Autodesk Fusion 360 part; units mm, degrees
(part 2 of 2)
fillet "Fillet2'" radius 0.5 4 edges at (74.2484, -13.991, 0.5) (60.2372, 0.0024, 0.5) (74.2484, 14.009, 0.5) (88.2372, 0.0024, 0.5) on bodies 7 in component "guards"
sketch "Sketch11" plane through (0, 0, 6) normal (0, 0, 1) x (-1, 0, 0)
  line L0 (-41.1231, -44.3731) -> (-33.1231, -44.3731)
  arc A0 (-33.1231, -45.8731) -> (-33.1231, -44.3731) centre (-33.1231, -45.1231) ccw
  line L1 (-33.1231, -45.8731) -> (-41.1231, -45.8731)
  arc A1 (-41.1231, -44.3731) -> (-41.1231, -45.8731) centre (-41.1231, -45.1231) ccw
  line L2 (-43.8731, -42.1231) -> (-43.8731, -32.1231)
  arc A2 (-42.3731, -32.1231) -> (-43.8731, -32.1231) centre (-43.1231, -32.1231) ccw
  line L3 (-42.3731, -32.1231) -> (-42.3731, -42.1231)
  arc A3 (-43.8731, -42.1231) -> (-42.3731, -42.1231) centre (-43.1231, -42.1231) ccw
  line L4 (-31.8731, -42.1231) -> (-31.8731, -32.1231)
  arc A4 (-30.3731, -32.1231) -> (-31.8731, -32.1231) centre (-31.1231, -32.1231) ccw
  line L5 (-30.3731, -32.1231) -> (-30.3731, -42.1231)
  arc A5 (-31.8731, -42.1231) -> (-30.3731, -42.1231) centre (-31.1231, -42.1231) ccw
  line L6 (-41.1231, -28.3731) -> (-33.1231, -28.3731)
  arc A6 (-33.1231, -29.8731) -> (-33.1231, -28.3731) centre (-33.1231, -29.1231) ccw
  line L7 (-33.1231, -29.8731) -> (-41.1231, -29.8731)
  arc A7 (-41.1231, -28.3731) -> (-41.1231, -29.8731) centre (-41.1231, -29.1231) ccw
  circle A8 centre (-45, -29.2462) radius 0.75
  circle A9 centre (-23.2462, -30.2462) radius 0.75
  circle A10 centre (-23.2462, -51) radius 0.75
  circle A11 centre (-51, -51) radius 0.75
  circle A12 centre (-45, -45) radius 0.75
  circle A13 centre (-23.2462, -44) radius 0.75
  circle A14 centre (-23.2462, -23.2462) radius 0.75
  circle A15 centre (-51, -30.2462) radius 0.75
  circle A16 centre (-44, -23.2462) radius 0.75
  circle A17 centre (-29.2462, -29.2462) radius 0.75
  circle A18 centre (-30.2462, -51) radius 0.75
  circle A19 centre (-51, -44) radius 0.75
  circle A20 centre (-44, -51) radius 0.75
  circle A21 centre (-29.2462, -45) radius 0.75
  circle A22 centre (-30.2462, -23.2462) radius 0.75
  circle A23 centre (-51, -23.2462) radius 0.75
  line L8 (-53.3731, -53.3731) -> (-20.8731, -53.3731)
  line L9 (-20.8731, -53.3731) -> (-20.8731, -20.8731)
  line L10 (-20.8731, -20.8731) -> (-53.3731, -20.8731)
  line L11 (-53.3731, -20.8731) -> (-53.3731, -53.3731)
  circle A24 centre (-51, -23.2462) radius 0.75
  circle A25 centre (-51, -51) radius 0.75
  circle A26 centre (-23.2462, -51) radius 0.75
  circle A27 centre (-23.2462, -23.2462) radius 0.75
  circle A28 centre (-23.2462, -23.2462) radius 1.5
  circle A29 centre (-51, -23.2462) radius 1.5
  circle A30 centre (-51, -51) radius 1.5
  circle A31 centre (-23.2462, -51) radius 1.5
  dimension "d111" = 3
  dimension "d112" = 3
  dimension "d113" = 3
  dimension "d114" = 3
  constraint concentric A23 A24
  constraint concentric A11 A25
  constraint concentric A10 A26
  constraint concentric A14 A27
  constraint concentric A27 A28
  constraint concentric A24 A29
  constraint concentric A25 A30
  constraint concentric A26 A31
  measures "d111" diameter of A28
  measures "d112" diameter of A29
  measures "d113" diameter of A30
  measures "d114" diameter of A31
extrude "Extrude1'''" add sketch "Sketch11" along normal blind 2 from surface at 10 separate body contours A8 | A9 | A12 | A13 | A15 | A16 | A17 | A18 | A19 | A20 | A21 | A22 | L8 L9 L10 L11 makes body 8 in component "platform2"
extrude "Extrude2'''" add sketch "Sketch11" along normal blind 1 from surface at 10 contours A28 | A29 | A30 | A31 bodies 8 in component "platform2"
extrude "Extrude1''''" add sketch "Sketch11" along normal blind 10 separate body contours A28 | A29 | A30 | A31 makes body 9 at (51.6843, 24.581, 9.3333) makes body 10 at (49.6827, 50.2826, 9.3333) makes body 11 at (21.7481, 23.321, 12.6667) makes body 12 at (21.9289, 50.2826, 9.3333) in component "posts"
sketch "Sketch12" plane through (0, 0, 18) normal (0, 0, 1) x (-1, 0, 0)
  arc A0 (-33.1231, -29.8731) -> (-33.1231, -28.3731) centre (-33.1231, -29.1231) ccw
  line L0 (-33.1231, -29.8731) -> (-41.1231, -29.8731)
  arc A1 (-41.1231, -28.3731) -> (-41.1231, -29.8731) centre (-41.1231, -29.1231) ccw
  line L1 (-41.1231, -28.3731) -> (-33.1231, -28.3731)
  arc A2 (-30.3731, -32.1231) -> (-31.8731, -32.1231) centre (-31.1231, -32.1231) ccw
  line L2 (-30.3731, -32.1231) -> (-30.3731, -42.1231)
  arc A3 (-31.8731, -42.1231) -> (-30.3731, -42.1231) centre (-31.1231, -42.1231) ccw
  line L3 (-31.8731, -42.1231) -> (-31.8731, -32.1231)
  arc A4 (-33.1231, -45.8731) -> (-33.1231, -44.3731) centre (-33.1231, -45.1231) ccw
  line L4 (-33.1231, -45.8731) -> (-41.1231, -45.8731)
  arc A5 (-41.1231, -44.3731) -> (-41.1231, -45.8731) centre (-41.1231, -45.1231) ccw
  line L5 (-41.1231, -44.3731) -> (-33.1231, -44.3731)
  arc A6 (-42.3731, -32.1231) -> (-43.8731, -32.1231) centre (-43.1231, -32.1231) ccw
  line L6 (-42.3731, -32.1231) -> (-42.3731, -42.1231)
  arc A7 (-43.8731, -42.1231) -> (-42.3731, -42.1231) centre (-43.1231, -42.1231) ccw
  line L7 (-43.8731, -42.1231) -> (-43.8731, -32.1231)
  circle A8 centre (-23.2462, -51) radius 1.5
  circle A9 centre (-23.2462, -23.2462) radius 1.5
  circle A10 centre (-51, -51) radius 1.5
  circle A11 centre (-51, -23.2462) radius 1.5
  line L8 (-53.3731, -20.8731) -> (-53.3731, -53.3731)
  line L9 (-53.3731, -53.3731) -> (-20.8731, -53.3731)
  line L10 (-20.8731, -53.3731) -> (-20.8731, -20.8731)
  line L11 (-20.8731, -20.8731) -> (-53.3731, -20.8731)
  line L12 (-41.1231, -23.9962) -> (-33.1231, -23.9962)
  arc A12 (-33.1231, -23.9962) -> (-33.1231, -22.4962) centre (-33.1231, -23.2462) ccw
  line L13 (-33.1231, -22.4962) -> (-41.1231, -22.4962)
  arc A13 (-41.1231, -22.4962) -> (-41.1231, -23.9962) centre (-41.1231, -23.2462) ccw
  line L14 (-41.1231, -23.2462) -> (-33.1231, -23.2462) construction
  line L15 (-51, -23.2462) -> (-51, -51)
  line L16 (-23.2462, -23.2462) -> (-23.2462, -51)
  line L17 (-48.5, -45.1231) -> (-48.5, -29.1231)
  arc A14 (-48.5, -29.1231) -> (-53.5, -29.1231) centre (-51, -29.1231) ccw
  line L18 (-53.5, -29.1231) -> (-53.5, -45.1231)
  arc A15 (-53.5, -45.1231) -> (-48.5, -45.1231) centre (-51, -45.1231) ccw
  line L19 (-51, -45.1231) -> (-51, -29.1231) construction
  line L20 (-20.7462, -45.1231) -> (-20.7462, -29.1231)
  arc A16 (-20.7462, -29.1231) -> (-25.7462, -29.1231) centre (-23.2462, -29.1231) ccw
  line L21 (-25.7462, -29.1231) -> (-25.7462, -45.1231)
  arc A17 (-25.7462, -45.1231) -> (-20.7462, -45.1231) centre (-23.2462, -45.1231) ccw
  line L22 (-23.2462, -45.1231) -> (-23.2462, -29.1231) construction
  line L23 (-23.2462, -47.6231) -> (-20.8731, -47.6231)
  line L24 (-23.2462, -26.6231) -> (-20.8731, -26.6231)
  line L25 (-51, -26.6231) -> (-53.3731, -26.6231)
  line L26 (-51, -47.6231) -> (-53.3731, -47.6231)
  line L27 (-37.1231, -32.5) -> (-36.5, -35)
  line L28 (-37.1231, -32.5) -> (-37.7462, -35)
  line L29 (-37.7462, -35) -> (-37.1231, -35)
  line L30 (-36.5, -35) -> (-37.1231, -35)
  point P0 (-51, -37.1231)
  point P1 (-23.2462, -37.1231)
  dimension "d125" = 1.5
  dimension "d126" = 5
  dimension "d127" = 5
  constraint tangent L12 A12
  constraint tangent A12 L13
  constraint parallel L12 L13
  constraint tangent L13 A13
  constraint tangent L12 A13
  constraint coincident A11.centre L15.start
  constraint coincident A10.centre L15.end
  constraint coincident A9.centre L16.start
  constraint coincident A8.centre L16.end
  constraint tangent L17 A14
  constraint tangent A14 L18
  constraint parallel L17 L18
  constraint tangent L18 A15
  constraint tangent L17 A15
  constraint parallel L15 L19
  constraint midpoint L15 P0
  constraint midpoint L19 P0
  constraint tangent L20 A16
  constraint tangent A16 L21
  constraint parallel L20 L21
  constraint tangent L21 A17
  constraint tangent L20 A17
  constraint parallel L16 L22
  constraint midpoint L16 P1
  constraint midpoint L22 P1
  constraint midpoint A17 L23.start
  constraint coincident L10 L23.end
  constraint tangent A17 L23
  constraint perpendicular L10 L23
  constraint midpoint A16 L24.start
  constraint coincident L10 L24.end
  constraint tangent A16 L24
  constraint perpendicular L10 L24
  constraint midpoint A14 L25.start
  constraint coincident L8 L25.end
  constraint tangent A14 L25
  constraint perpendicular L8 L25
  constraint midpoint A15 L26.start
  constraint coincident L8 L26.end
  constraint tangent A15 L26
  constraint perpendicular L8 L26
  measures "d125" diameter of A12
  measures "d126" diameter of A14
  measures "d127" diameter of A16
extrude "Extrude3'''" cut sketch "Sketch12" against normal blind 2 contours L8 A14 L25 | L8 L15 A14 A15 | L15 L17 A14 A15 | L10 A16 L24 | L8 A15 L26 | L10 L16 A16 A17 | L16 A16 L21 A17 | L10 A17 L23 | L12 A12 L13 A13 bodies 8 in component "platform2"
fillet "Fillet1''" radius 0.5 4 edges at (20.8731, 53.3731, 5) (53.3731, 53.3731, 5) (53.3731, 20.8731, 5) (20.8731, 20.8731, 5) on bodies 1
fillet "Fillet1'''" radius 0.5 4 edges at (20.8731, 53.3731, 17) (53.3731, 53.3731, 17) (53.3731, 20.8731, 17) (20.8731, 20.8731, 17) on bodies 8 in component "platform2"
fillet "Fillet2''" radius 0.5 4 edges at (53.3731, 26.6231, 17) (53.3731, 47.6231, 17) (20.8731, 47.6231, 17) (20.8731, 26.6231, 17) on bodies 8 in component "platform2"
extrude "Extrude4''" cut sketch "Sketch12" against normal blind 0.25 contours L27 L28 L29 L30 bodies 8 in component "platform2"
copy_body "CopyPasteBodies1" bodies 7 body 7 seen with x (1, 0, 0) y (0, 1, 0) z (0, 0, 1) at (-74.4635, -0.0203, -1.0542) makes body 13
copy_body "CopyPasteBodies1'" bodies 7 makes body 14 in component "guards"
move_body "Move1" bodies 14 to x (1, 0, 0) y (0, 1, 0) z (0, 0, 1) at (74.5, 0, 0) in component "guards"
copy_body "CopyPasteBodies3" bodies 7 makes body 15 in component "guards"
move_body "Move2" bodies 15 to x (1, 0, 0) y (0, 1, 0) z (0, 0, 1) at (0, 66, 0) in component "guards"
move_body "Move3" bodies 15 to x (1, 0, 0) y (0, 1, 0) z (0, 0, 1) at (0.2538, 8.2462, -8.5) in component "guards"
move_body "Move4" bodies 15 to x (1, 0, 0) y (0, 1, 0) z (0, 0, 1) at (0, 0, 9) in component "guards"
move_body "Move5'" bodies 15 to x (1, 0, 0) y (0, 1, 0) z (0, 0, 1) at (0, 0, -0.5) in component "guards"
copy_body "CopyPasteBodies4" bodies 15 makes body 16 in component "guards"
move_body "Move6'" bodies 16 to x (1, 0, 0) y (0, 1, 0) z (0, 0, 1) at (74.5, 0, 0) in component "guards"
component "arms" placed x (1, 0, 0) y (0, 1, 0) z (0, 0, 1) at (0.0365, -0.0203, -1.0542)
component "platform2" placed x (1, 0, 0) y (0, 1, 0) z (0, 0, 1) at (0, 0, 0)
component "posts" placed x (1, 0, 0) y (0, 1, 0) z (0, 0, 1) at (0, 0, 0)
component "guards" placed x (1, 0, 0) y (0, 1, 0) z (0, 0, 1) at (-74.4635, -0.0203, -1.0542)
named bodies: "Body3", "Body3 (1)"
